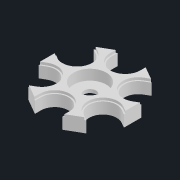
# Autodesk Inventor part: motor15
Saved by Autodesk Inventor 2022.2 (Build 262287010, 287A)
## iProperties
Created: 2023-07-17
Part Number: motor15
Material: Generic
Document SubType Name: Modeling
Designer: StijnC
Density: 1 g/cm^3
Appearance: Default
Author: StijnC
## iProperties of the stored document motor_3DPrint.ipt
Created: 2023-07-17
Part Number: motor_3DPrint
Material: Generic
Document SubType Name: Modeling
Designer: StijnC
Density: 1 g/cm^3
Appearance: Default
Author: StijnC
Autodesk Inventor part; units mm, degrees
ref_plane "YZ Plane" through (0, 0, 0) normal (1, 0, 0) x (0, 1, 0)
ref_plane "XZ Plane" through (0, 0, 0) normal (0, 1, 0) x (-1, 0, 0)
ref_plane "XY Plane" through (0, 0, 0) normal (0, 0, 1) x (1, 0, 0)
sketch "Sketch1" plane through (0, 0, 0) normal (0, 1, 0) x (-1, 0, 0)
  circle A0 centre (0, 0) radius 30
  circle A1 centre (0, 20.5) radius 8.75
  circle A2 centre (-17.7535, 10.25) radius 8.75
  circle A3 centre (-17.7535, -10.25) radius 8.75
  circle A4 centre (0, -20.5) radius 8.75
  circle A5 centre (17.7535, -10.25) radius 8.75
  circle A6 centre (17.7535, 10.25) radius 8.75
  circle A7 centre (20.5, 0) radius 7.5
  circle A8 centre (14.4957, 14.4957) radius 7.5
  circle A9 centre (0, 20.5) radius 7.5
  circle A10 centre (-14.4957, 14.4957) radius 7.5
  circle A11 centre (-20.5, 0) radius 7.5
  circle A12 centre (-14.4957, -14.4957) radius 7.5
  circle A13 centre (0, -20.5) radius 7.5
  circle A14 centre (14.4957, -14.4957) radius 7.5
  dimension "d0" = 60
  dimension "d19" = 17.5
  dimension "d20" = 20.5
  dimension "d23" = 360
  dimension "d25" = 15
  dimension "d26" = 20.5
  dimension "d29" = 360
  constraints: 15 centre point, 1 coincident, 1 horizontal alignment, 1 vertical alignment, 30 other
  measures "d0" diameter of A0
  measures "d19" diameter of A1
  measures "d20" distance of point (0, 0) A1.centre
  measures "d25" diameter of A7
  measures "d26" distance of point (0, 0) A7.centre
extrude "Extrusion1" add sketch "Sketch1" along normal blind 8 contours A0 | A1 A8 A10 | A10 A1 | A1 A10 A2 | A8 A6 A1 | A1 A8 | A1 A8 A6 A7 A5 A14 A4 A12 A3 A11 A2 A10 | A10 A2 A11 | A2 A10 | A8 A6 | A6 A7 A8 | A11 A2 | A2 A11 A3 | A11 A3 A12 | A3 A11 | A7 A6 | A6 A7 A5 | A12 A3 | A3 A12 A4 | A7 A5 A14 | A5 A7 | A12 A4 A14 | A4 A12 | A14 A5 | A5 A14 A4 | A4 A14 | A9 | A13
sketch "Sketch2" plane through (0, 8, 0) normal (0, 1, 0) x (1, 0, 0)
  circle A0 centre (0, -20.5) radius 8.75
  line L0 (-8.75, -20.5) -> (-8.75, -28.6956)
  line L1 (8.75, -20.5) -> (8.75, -28.6956)
  circle A1 centre (0, 0) radius 30 projected
  dimension "d3" = 17.5
  dimension "d4" = 20.5
  constraints: 4 end point, 4 point on circle, 2 tangent, 2 vertical, 1 centre point, 1 vertical alignment
  measures "d3" diameter of A0
  measures "d4" distance of point (0, 0) A0.centre
extrude "Extrusion2" cut sketch "Sketch2" against normal blind 1.4 contours A0 | L1 A1 L0 A0 picked at (-5.5585, -28.7503)
sketch "Sketch3" plane through (0, 6.6, 20.5) normal (0, 1, 0) x (-1, 0, 0)
  arc A0 (-8.75, 0) -> (8.75, 0) centre (0, 0) ccw projected
  circle A1 centre (0, 0) radius 8
  line L0 (8, 0) -> (8, 8.4137)
  line L1 (-8, 0) -> (-8, 8.4137)
  arc A2 (8.75, 8.1956) -> (-8.75, 8.1956) centre (0, -20.5) ccw projected
  dimension "d7" = 16
  constraints: 4 end point, 4 point on circle, 2 tangent, 2 vertical, 1 centre point, 1 coincident
  measures "d7" diameter of A1
extrude "Extrusion3" cut sketch "Sketch3" against normal through all
pattern_circular "Circular Pattern1" count 6 over 360 about axis through (0, 0, 0) along (0, 1, 0) of "Extrusion2", "Extrusion3"
sketch "Sketch7" plane through (0, 8, 0) normal (0, 1, 0) x (1, 0, 0)
  arc A0 (8, -20.5) -> (-8, -20.5) centre (0, -20.5) ccw projected
  circle A1 centre (0, -20.5) radius 8.75
  arc A2 (-13.7535, -17.1782) -> (-21.7535, -3.3218) centre (-17.7535, -10.25) ccw projected
  circle A3 centre (-17.7535, -10.25) radius 8.75
  line L0 (-21.04, -21.385) -> (-13.7535, -17.1782) projected
  line L1 (-8, -28.9137) -> (-8, -20.5) projected
  line L2 (-8, -24.0444) -> (-16.823, -18.9504)
  arc A4 (-20.4761, -21.9255) -> (-8.75, -28.6956) centre (0, 0) ccw projected
  arc A5 (-21.04, -21.385) -> (-20.4761, -21.9255) centre (0, 0) ccw projected
  arc A6 (-8.75, -28.6956) -> (-8, -28.9137) centre (0, 0) ccw projected
  dimension "d32" = 17.5
  dimension "d33" = 17.5
  constraints: 2 coincident, 2 end point, 2 point on line, 6 other
extrude "Extrusion6" cut sketch "Sketch7" against normal blind 10 contours L1 A6 A4 A5 L0 L2
pattern_circular "Circular Pattern2" count 6 over 360 about axis through (0, -10, 0) along (0, 1, 0) of "Extrusion6"
sketch "Sketch4" plane through (0, 8, 0) normal (0, 1, 0) x (1, 0, 0)
  circle A0 centre (0, 0) radius 3.5
  dimension "d13" = 7
  constraints: 1 centre point, 1 coincident
  measures "d13" diameter of A0
extrude "Extrusion4" cut sketch "Sketch4" against normal through all
sketch "Sketch8" plane through (0, 8, 0) normal (0, 1, 0) x (1, 0, 0)
  circle A0 centre (0, 0) radius 9.5
  dimension "d39" = 19
  constraints: 1 centre point, 1 coincident
  measures "d39" diameter of A0
extrude "Extrusion7" cut sketch "Sketch8" against normal blind 6
equation "\"d26\" = d20"
equation "\"d4\" = d20"
body "Solid1"
